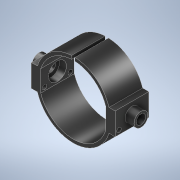
# Autodesk Inventor part: Soporte_PVC_Balancin
Saved by Autodesk Inventor 2022 (Build 260153000, 153)
## iProperties
Created: 2022-02-24
Part Number: Soporte_PVC_Balancin
Material: Generic
Document SubType Name: Modeling
Designer: hurta
Density: 1 g/cm^3
Appearance: Glossy - Black
Author: hurta
Autodesk Inventor part; units mm, degrees
ref_plane "XZ Plane" through (0, 0, 0) normal (0, 1, 0) x (-1, 0, 0)
ref_plane "XY Plane" through (0, 0, 0) normal (0, 0, 1) x (1, 0, 0)
sketch "Sketch1" plane through (0, 0, 0) normal (0, 0, 1) x (1, 0, 0)
  circle A0 centre (0, 0) radius 30.5
  circle A1 centre (0, 0) radius 33.5
  dimension "d0" = 61
  dimension "d1" = 67
  constraints: 2 centre point, 2 coincident
  measures "d0" diameter of A0
  measures "d1" diameter of A1
extrude "Extrusion1" add sketch "Sketch1" along normal mid plane 30
ref_plane "Work Plane2" through (-33.5, 0, 0) normal (1, 0, 0) x (0, 1, 0)
ref_plane "Work Plane1" through (33.5, 0, 0) normal (1, 0, 0) x (0, 1, 0)
sketch "Sketch3" plane through (33.5, 0, 0) normal (1, 0, 0) x (0, 1, 0)
  line L0 (-30.5, 15) -> (30.5, 15) projected
  line L1 (-10, -15) -> (10, -15)
  line L2 (10, -15) -> (10, 15)
  line L3 (10, 15) -> (-10, 15)
  line L4 (-10, 15) -> (-10, -15)
  line L5 (-10, -15) -> (10, 15) construction
  line L6 (10, -15) -> (-10, 15) construction
  point P0 (0, 0)
  dimension "d20" = 20
  constraints: 12 end point, 2 midpoint, 2 parallel, 1 horizontal, 1 perpendicular, 1 point on line
  measures "d20" distance between parallel lines of L4 L2
extrude "Extrusion2" add sketch "Sketch3" along normal blind 4 and the other way blind 4.5
sketch "Sketch4" plane through (-33.5, 0, 0) normal (1, 0, 0) x (0, 1, 0)
  line L0 (30.5, -15) -> (-30.5, -15) projected
  line L1 (10, 15) -> (-10, 15)
  line L2 (-10, 15) -> (-10, -15)
  line L3 (-10, -15) -> (10, -15)
  line L4 (10, -15) -> (10, 15)
  line L5 (10, 15) -> (-10, -15) construction
  line L6 (-10, 15) -> (10, -15) construction
  point P0 (0, 0)
  dimension "d25" = 20
  constraints: 12 end point, 2 midpoint, 2 parallel, 1 horizontal, 1 perpendicular, 1 point on line
  measures "d25" distance between parallel lines of L2 L4
extrude "Extrusion3" add sketch "Sketch4" along normal blind 4.5 and the other way blind 4
sketch "Sketch5" plane through (33.5, 0, 0) normal (1, 0, 0) x (0, 1, 0)
  circle A0 centre (0, 0) radius 3.5
  circle A1 centre (0, 0) radius 6.25
  dimension "d30" = 7
  dimension "d31" = 12.5
  constraints: 2 centre point, 2 coincident
  measures "d30" diameter of A0
  measures "d31" diameter of A1
extrude "Extrusion4" add sketch "Sketch5" along normal blind 12
sketch "Sketch6" plane through (-37.5, 0, 0) normal (-1, 0, 0) x (0, 0, 1)
  circle A0 centre (0, 0) radius 3.5
  circle A1 centre (0, 0) radius 6.25
  dimension "d35" = 7
  dimension "d36" = 12.5
  constraints: 2 centre point, 2 coincident
  measures "d35" diameter of A0
  measures "d36" diameter of A1
extrude "Extrusion5" add sketch "Sketch6" along normal blind 8
sketch "Sketch8" plane through (-29, 0, 0) normal (1, 0, 0) x (0, 0, -1)
  point P0 (0, 0)
  point P1 (0, 0)
  constraints: 1 coincident
hole "Hole3" at (-29, 0, 0) direction (-1, 0, 0) diameter 8.4 depth 16.5 counterbore diameter 16 counterbore depth 6.15
sketch "Sketch9" plane through (29, 0, 0) normal (-1, 0, 0) x (0, 0, 1)
  point P0 (0, 0)
  point P1 (0, 0)
  constraints: 1 coincident
hole "Hole4" at (29, 0, 0) direction (1, 0, 0) diameter 8.4 depth 16.5 counterbore diameter 16 counterbore depth 6.15
sketch "Sketch10" plane through (-37.5, 0, 0) normal (-1, 0, 0) x (0, 0, 1)
  line L0 (-15, 10) -> (-15, -10) projected
  line L1 (15, -10) -> (15, 10) projected
  line L2 (-15, -10) -> (15, -10) projected
  point P0 (0, 0)
  point P1 (11.5, -6.5)
  point P2 (-11.5, -6.5)
  dimension "d58" = 3.5
  dimension "d59" = 3.5
  dimension "d60" = 3.5
  constraints: 1 horizontal alignment
  measures "d58" distance from line of point (-11.5, -6.5) L0
  measures "d59" distance from line of point (11.5, -6.5) L1
  measures "d60" distance from line of point (-11.5, -6.5) L2
hole "Hole5" at (-37.5, -6.5, 11.5) at (-37.5, -6.5, -11.5) direction (1, 0, 0) diameter 4.134 depth 75 thread size "M5x0.8" class "6H" standard "ANSI Metric M Profile"
sketch "Sketch11" plane through (0, 0, 15) normal (0, 0, 1) x (1, 0, 0)
  line L0 (-1.5, 37.1959) -> (1.5, 37.1959)
  line L1 (1.5, 37.1959) -> (1.5, 23.2844)
  line L2 (1.5, 23.2844) -> (-1.5, 23.2844)
  line L3 (-1.5, 23.2844) -> (-1.5, 37.1959)
  point P0 (0, 0)
  dimension "d68" = 1.5
  dimension "d69" = 1.5
  constraints: 8 end point, 2 parallel, 1 horizontal, 1 perpendicular
  measures "d68" distance from line of point (0, 0) L1
  measures "d69" distance from line of point (0, 0) L3
extrude "Extrusion7" cut sketch "Sketch11" against normal through all
equation "\"d25\" = d20"
equation "\"d59\" = d58"
body "Solid1"
